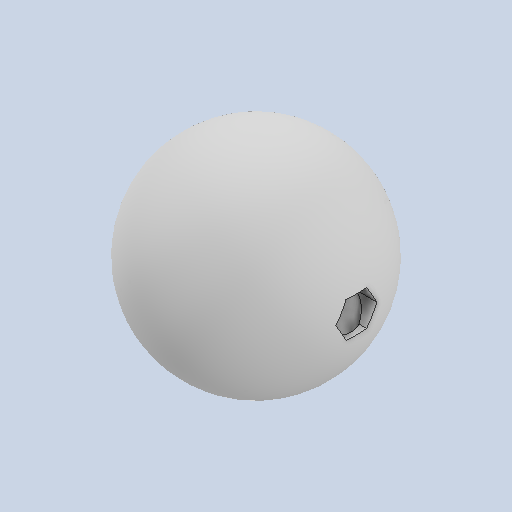
# Autodesk Inventor part: peca_008_001
Saved by Autodesk Inventor 2026 (Build 300175000, 175)
## iProperties
Created: 2025-03-26
Part Number: peca_008_001
Material: Generic
Document SubType Name: Modeling
Designer: Carlos Dias
Density: 1 g/cm^3
Appearance: Default
Author: Carlos Dias
Autodesk Inventor part; units mm, degrees
ref_plane "YZ Plane" through (0, 0, 0) normal (1, 0, 0) x (0, 1, 0)
ref_plane "XZ Plane" through (0, 0, 0) normal (0, 1, 0) x (-1, 0, 0)
ref_plane "XY Plane" through (0, 0, 0) normal (0, 0, 1) x (1, 0, 0)
sketch "Sketch1" plane through (0, 0, 0) normal (0, 0, 1) x (1, 0, 0)
  arc A0 (0, 5) -> (0, -5) centre (0, 0) ccw
  arc A1 (0, 10) -> (0, -10) centre (0, 0) ccw
  line L0 (0, 10) -> (0, 5)
  line L1 (0, -5) -> (0, -10)
  dimension "d0" = 5
  dimension "d1" = 10
  constraints: 4 end point, 4 point on circle, 4 vertical alignment, 3 coincident, 2 centre point, 1 collinear, 1 vertical
  measures "d0" radius of A0
  measures "d1" radius of A1
revolve "Revolution1" add sketch "Sketch1" angle 360 about axis through (0, 10, 0) along (0, -1, 0)
sketch "Sketch2" plane through (0, 0, 0) normal (1, 0, 0) x (0, 1, 0)
  circle A0 centre (7.5, 0) radius 2
  line L0 (0, -10) -> (0, 10)
  point P0 (0, 0)
  point P1 (0, 0)
  dimension "d3" = 4
  dimension "d4" = 7.5
  dimension "d5" = 20
  constraints: 2 coincident, 2 end point, 1 centre point, 1 horizontal alignment, 1 midpoint, 1 vertical
  measures "d3" diameter of A0
  measures "d4" distance of point (0, 0) A0.centre
  measures "d5" distance of L0.start L0.end
revolve "Revolution2" cut sketch "Sketch2" angle 360 about axis through (0, 0, -10) along (0, 0, -1)
sketch "Sketch3" plane through (0, 0, 0) normal (1, 0, 0) x (0, 1, 0)
  line L0 (-1.7321, 1) -> (0, 2)
  line L1 (0, 2) -> (1.7321, 1)
  line L2 (1.7321, 1) -> (1.7321, -1)
  line L3 (1.7321, -1) -> (0, -2)
  line L4 (0, -2) -> (-1.7321, -1)
  line L5 (-1.7321, -1) -> (-1.7321, 1)
  point P0 (0, 0)
  point P1 (0, 0)
  point P2 (1.7321, 0)
  dimension "d10" = 2
  constraints: 12 end point, 2 coincident, 1 horizontal alignment, 1 midpoint, 13 other
  measures "d10" distance of L2.end L3.end
extrude "Extrusion1" cut sketch "Sketch3" along normal through all both and the other way through all
body "Solid1"
